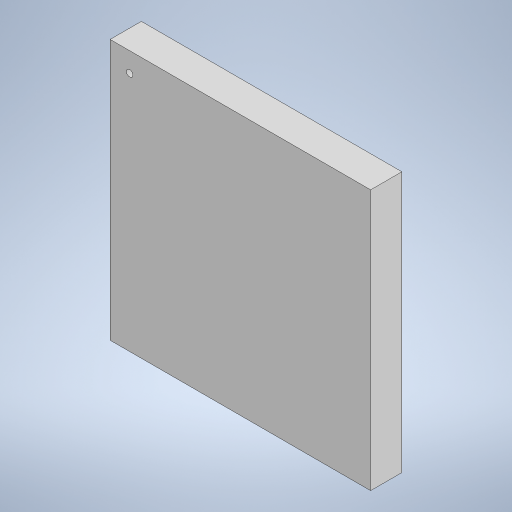
# Autodesk Inventor part: H mustek
Saved by Autodesk Inventor 2023 (Build 270158000, 158)
## iProperties
Created: 2023-01-20
Part Number: H mustek
Material: Všeobecné
Document SubType Name: Modeling
Designer: Kuba
Mass: 0.959529 g
Surface Area: 9.95377 cm^2
Volume: 0.959529 cm^3
Density: 1 g/cm^3
Appearance: Výchozí
Author: Kuba
Autodesk Inventor part; units mm, degrees
ref_plane "YZ Plane" through (0, 0, 0) normal (1, 0, 0) x (0, 1, 0)
ref_plane "XZ Plane" through (0, 0, 0) normal (0, 1, 0) x (-1, 0, 0)
ref_plane "XY Plane" through (0, 0, 0) normal (0, 0, 1) x (1, 0, 0)
sketch "Náčrt1" plane through (0, 0, 0) normal (0, 0, 1) x (1, 0, 0)
  line L0 (0, 0) -> (-10, 0) construction
  line L1 (-10, 0) -> (-10, -10) construction
  line L2 (-10, -10) -> (0, -10) construction
  line L3 (0, -10) -> (0, 0) construction
  line L4 (-10, -10) -> (10, -10)
  line L5 (10, -10) -> (10, 10)
  line L6 (10, 10) -> (-10, 10)
  line L7 (-10, 10) -> (-10, -10)
  dimension "d0" = 10
  dimension "d1" = 10
  dimension "d2" = 20
  dimension "d3" = 20
  constraints: 16 end point, 4 parallel, 2 horizontal, 2 perpendicular
  measures "d0" distance of L2.end L1.end
  measures "d1" distance of L1.end L0.end
  measures "d2" distance of L6.end L5.end
  measures "d3" distance of L5.end L4.end
extrude "Vysunutí1" add sketch "Náčrt1" along normal blind 2.4
sketch "Náčrt3" plane through (0, 0, 2.4) normal (0, 0, 1) x (1, 0, 0)
  line L0 (-10, 10) -> (-10, -10) projected
  line L1 (10, 10) -> (-10, 10) projected
  point P0 (0, 0)
  point P1 (-8.5, 8.5)
  dimension "d12" = 1.5
  dimension "d13" = 1.5
  measures "d12" distance from line of L0 point (-8.5, 8.5)
  measures "d13" distance from line of L1 point (-8.5, 8.5)
hole "Díra1" at (-8.5, 8.5, 2.4) direction (0, 0, -1) diameter 0.5 end through all
